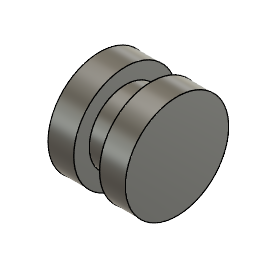
part 2 (12) (Autodesk Fusion 360 design; units mm, degrees)
part number: 2026-06-23-23-08-20-307
Autodesk Fusion 360 part; units mm, degrees
sketch "Sketch1" plane through (0, 0, 0) normal (0, 1, 0) x (1, 0, 0)
  line L0 (0, 0) -> (0, -50)
  line L1 (0, -50) -> (-25, -50)
  line L2 (-50, -50) -> (-75, -50)
  line L3 (-75, -50) -> (-75, -25)
  line L4 (-75, -25) -> (-95, -15)
  line L5 (-95, -15) -> (-95, 0)
  line L6 (-95, 0) -> (0, 0)
  line L7 (-25, -50) -> (-25, -35)
  line L8 (-25, -35) -> (-50, -35)
  line L9 (-50, -35) -> (-50, -50)
  constraint coincident L0.start L6.end
  constraint vertical L0
  constraint perpendicular L0 L1
  constraint perpendicular L2 L3
  constraint perpendicular L2 L5
  constraint perpendicular L0 L6
  constraint perpendicular L1 L7
  constraint perpendicular L7 L8
  constraint perpendicular L2 L9
revolve "Revolve1" add sketch "Sketch1" angle 360 about axis through (-95, 0, 0) along (1, 0, 0)
